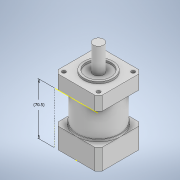
# Autodesk Inventor part: Gearbox
Saved by Autodesk Inventor 2021 (Build 250183000, 183)
## iProperties
Created: 2021-10-06
Part Number: Gearbox
Material: Generic
Document SubType Name: Modeling
Designer: nxf77172
Density: 3.02523 g/cm^3
Appearance: Default
Mass: 856 g
Surface Area: 313.194 cm^2
Volume: 282.954 cm^3
Author: nxf77172
Autodesk Inventor part; units mm, degrees
ref_plane "YZ Plane" through (0, 0, 0) normal (1, 0, 0) x (0, 1, 0)
ref_plane "XZ Plane" through (0, 0, 0) normal (0, 1, 0) x (-1, 0, 0)
ref_plane "XY Plane" through (0, 0, 0) normal (0, 0, 1) x (1, 0, 0)
sketch "Sketch1" plane through (0, 0, 0) normal (0, 1, 0) x (-1, 0, 0)
  line L0 (30, 30) -> (-30, 30)
  line L1 (-30, 30) -> (-30, -30)
  line L2 (-30, -30) -> (30, -30)
  line L3 (30, -30) -> (30, 30)
  line L4 (30, 30) -> (-30, -30) construction
  line L5 (-30, 30) -> (30, -30) construction
  circle A0 centre (0, 0) radius 29
  circle A1 centre (0, 0) radius 30
  point P0 (0, 0)
  dimension "d0" = 60
  dimension "d1" = 60
  dimension "d2" = 58
  constraints: 12 end point, 3 coincident, 2 centre point, 2 midpoint, 2 parallel, 1 horizontal, 1 perpendicular, 1 tangent
  measures "d0" distance of L0.end L1.end
  measures "d1" distance of L0.start L0.end
  measures "d2" diameter of A0
extrude "Extrusion1" add sketch "Sketch1" along normal blind 28 contours L3 A1 L0 | A1 L1 L0 | A1 | L3 L2 A1 | A1 L2 L1 | A0
sketch "Sketch2" plane through (0, 28, 0) normal (0, 1, 0) x (1, 0, 0)
  circle A0 centre (0, 0) radius 30
  constraints: 1 centre point, 1 coincident
extrude "Extrusion2" add sketch "Sketch2" along normal blind 3
sketch "Sketch3" plane through (0, 31, 0) normal (0, 1, 0) x (1, 0, 0)
  circle A0 centre (0, 0) radius 29
  dimension "d7" = 58
  constraints: 1 centre point, 1 coincident
  measures "d7" diameter of A0
extrude "Extrusion3" add sketch "Sketch3" along normal blind 39.5
sketch "Sketch4" plane through (0, 70.5, 0) normal (0, 1, 0) x (1, 0, 0)
  line L0 (-30, -30) -> (30, -30) projected
  line L1 (30, -30) -> (30, 30) projected
  line L2 (-30, -30) -> (30, -30)
  line L3 (30, -30) -> (30, 30)
  line L4 (30, 30) -> (-30, 30)
  line L5 (-30, 30) -> (-30, -30)
  line L6 (30, 30) -> (-30, 30) construction
  line L7 (-30, -30) -> (30, 30) construction
  line L8 (30, -30) -> (-30, 30) construction
  circle A0 centre (-23.575, -23.575) radius 2.5
  circle A1 centre (-23.575, 23.575) radius 2.5
  circle A2 centre (23.575, 23.575) radius 2.5
  circle A3 centre (23.575, -23.575) radius 2.5
  line L9 (-23.575, -23.575) -> (-23.575, 23.575) construction
  point P0 (0, 0)
  dimension "d10" = 5
  dimension "d11" = 5
  dimension "d12" = 47.15
  dimension "d13" = 5
  dimension "d14" = 5
  dimension "d15" = 47.15
  dimension "d16" = 47.15
  dimension "d17" = 47.15
  constraints: 14 end point, 5 point on line, 4 centre point, 3 parallel, 1 horizontal, 1 perpendicular
  measures "d10" diameter of A0
  measures "d11" diameter of A1
  measures "d12" distance of L9.end L9.start
  measures "d13" diameter of A2
  measures "d14" diameter of A3
  measures "d15" distance of A2.centre L9.end
  measures "d16" distance of A3.centre A2.centre
  measures "d17" distance of A3.centre L9.start
sketch "Sketch5" plane through (-30, 0, 30) normal (0, 0, 1) x (1, 0, 0)
  line L0 (0, 0) -> (0, 28) construction
  line L1 (0, 70.5) -> (0, 0) construction
  line L2 (59, 70.5) -> (1, 70.5) projected
  point P0 (30, 0)
  dimension "d21" = 70.5
  constraints: 2 end point, 1 collinear, 1 point on line
  measures "d21" distance of L1.start L0.start
extrude "Extrusion4" add sketch "Sketch4" along normal blind 19
sketch "Sketch6" plane through (0, 89.5, 0) normal (0, 1, 0) x (1, 0, 0)
  circle A0 centre (0, 0) radius 20
  circle A1 centre (0, 0) radius 17
  circle A2 centre (0, 0) radius 7
  dimension "d22" = 14
  dimension "d23" = 40
  dimension "d24" = 3
  constraints: 3 centre point, 3 coincident
  measures "d22" diameter of A2
  measures "d23" diameter of A0
  measures "d24" radial gap between concentric circles of A0 A1
extrude "Extrusion5" add sketch "Sketch6" along normal blind 2.5 contours A0
sketch "Sketch7" plane through (0, 89.5, 0) normal (0, 1, 0) x (1, 0, 0)
  circle A0 centre (0, 0) radius 7
  dimension "d27" = 14
  constraints: 1 centre point, 1 coincident
  measures "d27" diameter of A0
extrude "Extrusion6" add sketch "Sketch7" along normal blind 35
chamfer "Chamfer1" distance 5 angle 45 8 edges at (-30, 80, 30) (30, 80, 30) (-30, 14, 30) (30, 14, 30) (30, 80, -30) (-30, 80, -30) (-30, 14, -30) (30, 14, -30)
sketch "Sketch8" plane through (0, 0, 0) normal (0, -1, 0) x (1, 0, 0)
  circle A0 centre (0, 0) radius 4
  dimension "d33" = 8
  constraints: 1 centre point, 1 coincident
  measures "d33" diameter of A0
extrude "Extrusion7" cut sketch "Sketch8" against normal blind 30
equation "\"d1\" = d0"
equation "\"d15\" = d12"
equation "\"d16\" = d12"
equation "\"d17\" = d12"
body "Solid1"
